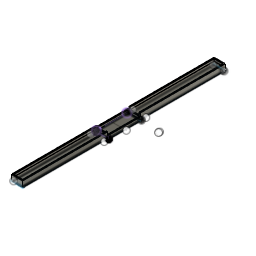
BitHolder (Autodesk Fusion 360 design; units mm, degrees)
Autodesk Fusion 360 part; units mm, degrees
sketch "Sketch2" plane through (0, 0, 0) normal (0, 0, 1) x (1, 0, 0)
  line L0 (0, 0) -> (25.146, 0)
  line L1 (25.146, 0) -> (25.146, 68.58)
  line L2 (25.146, 68.58) -> (0, 68.58)
  line L3 (0, 68.58) -> (0, 0)
  line L4 (0, 68.58) -> (-2.54, 68.58)
  line L5 (-2.54, 68.58) -> (-2.54, 0)
  line L6 (-2.54, 0) -> (0, 0)
  line L7 (0, 0) -> (0, 68.58)
  line L8 (25.146, 0) -> (27.686, 0)
  line L9 (27.686, 0) -> (27.686, 68.58)
  line L10 (27.686, 68.58) -> (25.146, 68.58)
  line L11 (25.146, 68.58) -> (25.146, 0)
  line L12 (71.12, 68.58) -> (71.12, 66.04)
  line L13 (-2.54, 66.04) -> (-2.54, 68.58)
  line L14 (-2.54, 68.58) -> (27.686, 68.58)
  line L15 (27.686, 68.58) -> (27.686, 71.12)
  line L16 (27.686, 71.12) -> (-2.54, 71.12)
  line L17 (-2.54, 71.12) -> (-2.54, 68.58)
  line L18 (27.686, 0) -> (-2.54, 0)
  line L19 (-2.54, 0) -> (-2.54, -2.54)
  line L20 (-2.54, -2.54) -> (27.686, -2.54)
  line L21 (27.686, -2.54) -> (27.686, 0)
  dimension "d46" = 25.146
  dimension "d47" = 68.58
  dimension "d48" = 2.54
  dimension "d49" = 2.54
  dimension "d51" = 2.54
  dimension "d52" = 2.54
  dimension "d53" = 30.226
  dimension "d54" = 2.54
  dimension "d55" = 30.226
  constraint horizontal L0
  constraint vertical L1
  constraint horizontal L2
  constraint vertical L3
  constraint coincident L0.start L3.end
  constraint horizontal L4
  constraint vertical L5
  constraint horizontal L6
  constraint vertical L7
  constraint horizontal L8
  constraint vertical L9
  constraint horizontal L10
  constraint vertical L11
  constraint vertical L12
  constraint vertical L13
  constraint horizontal L14
  constraint vertical L15
  constraint horizontal L16
  constraint vertical L17
  constraint horizontal L18
  constraint vertical L19
  constraint horizontal L20
  constraint vertical L21
  measures "d46" distance of L1.end L2.end
  measures "d47" distance of L0.start L2.end
  measures "d48" distance of L2.end L4.end
  measures "d49" distance of L9.end L1.end
  measures "d51" distance of L4.end L13.start
  measures "d52" distance of L4.end L16.end
  measures "d53" distance of L8.end L5.end
  measures "d54" distance of L5.end L19.end
  measures "d55" distance of L15.end L16.end
extrude "Extrude10" add sketch "Sketch2" along normal blind 2.54 contours L0 L1 L2 L3 L7 L11 L14 L18 makes body 1
extrude "Extrude11" add sketch "Sketch2" along normal blind 7.62 contours L1 L8 L9 L10 L11 L14 L18 bodies 1
extrude "Extrude12" add sketch "Sketch2" along normal blind 7.62 contours L0 L6 L8 L18 L19 L20 L21 bodies 1
extrude "Extrude13" add sketch "Sketch2" along normal blind 7.62 contours L3 L4 L5 L6 L7 L13 L14 L18 bodies 1
extrude "Extrude14" add sketch "Sketch2" along normal blind 7.62 contours L2 L4 L10 L14 L15 L16 L17 bodies 1
sketch "Sketch3" plane through (0, 0, 0) normal (0, 0, 1) x (1, 0, 0)
  line L0 (2.573, -2.54) -> (22.573, -2.54)
  line L1 (22.573, -2.54) -> (22.573, -191.036)
  line L2 (22.573, -191.036) -> (2.573, -191.036)
  line L3 (2.573, -191.036) -> (2.573, -2.54)
  line L4 (-2.54, -2.54) -> (27.686, -2.54)
  line L5 (27.686, -2.54) -> (27.686, -12.7) construction
  line L6 (-2.54, -2.54) -> (-2.54, -13.5317) construction
  line L7 (2.573, -2.54) -> (0.033, -2.54) construction
  line L8 (0.033, -191.036) -> (2.573, -191.036) construction
  line L9 (2.573, -2.54) -> (0.033, -2.54)
  line L10 (0.033, -2.54) -> (0.033, -191.036)
  line L11 (0.033, -191.036) -> (2.573, -191.036)
  line L12 (2.573, -191.036) -> (2.573, -2.54)
  line L13 (22.573, -2.54) -> (25.113, -2.54)
  line L14 (25.113, -2.54) -> (25.113, -191.036)
  line L15 (25.113, -191.036) -> (22.573, -191.036)
  line L16 (22.573, -191.036) -> (22.573, -2.54)
  line L17 (0.033, -191.036) -> (25.113, -191.036)
  line L18 (25.113, -191.036) -> (25.113, -193.576)
  line L19 (25.113, -193.576) -> (0.033, -193.576)
  line L20 (0.033, -193.576) -> (0.033, -191.036)
  line L21 (-2.54, 68.58) -> (-2.54, 0)
  line L22 (-2.54, 34.29) -> (30.48, 34.29)
  line L23 (25.113, 71.12) -> (25.113, 259.616)
  line L24 (22.573, 259.616) -> (22.573, 71.12)
  line L25 (2.573, 259.616) -> (2.573, 71.12)
  line L26 (0.033, 71.12) -> (0.033, 259.616)
  line L27 (2.573, 71.12) -> (22.573, 71.12)
  line L28 (2.573, 71.12) -> (0.033, 71.12)
  line L29 (22.573, 71.12) -> (25.113, 71.12)
  line L30 (27.686, 71.12) -> (27.686, 81.28) construction
  line L31 (-2.54, 71.12) -> (-2.54, 82.1117) construction
  line L32 (25.113, 262.156) -> (0.033, 262.156)
  line L33 (0.033, 259.616) -> (2.573, 259.616)
  line L34 (22.573, 259.616) -> (2.573, 259.616)
  line L35 (25.113, 259.616) -> (22.573, 259.616)
  line L36 (25.113, 259.616) -> (25.113, 262.156)
  line L37 (0.033, 262.156) -> (0.033, 259.616)
  dimension "d66" = 188.496
  dimension "d67" = 20
  dimension "d68" = 5.113
  dimension "d69" = 5.113
  dimension "d71" = 188.496
  dimension "d72" = 2.54
  dimension "d73" = 188.496
  dimension "d74" = 2.54
  dimension "d75" = 188.496
  dimension "d76" = 25.08
  dimension "d77" = 2.54
  constraint horizontal L0
  constraint vertical L1
  constraint horizontal L2
  constraint vertical L3
  constraint coincident L0.start L4
  constraint coincident L4.end L5.start
  constraint perpendicular L4 L5
  constraint coincident L4.start L6.start
  constraint perpendicular L4 L6
  constraint horizontal L7
  constraint horizontal L8
  constraint horizontal L9
  constraint vertical L10
  constraint horizontal L11
  constraint vertical L12
  constraint horizontal L13
  constraint vertical L14
  constraint horizontal L15
  constraint vertical L16
  constraint horizontal L17
  constraint vertical L18
  constraint horizontal L19
  constraint vertical L20
  constraint midpoint L21 L22.start
  constraint perpendicular L6 L22
  constraint symmetric L0.start L22 L25.end
  constraint symmetric L0.end L22 L24.end
  constraint symmetric L1.end L22 L24.start
  constraint symmetric L2.end L22 L25.start
  constraint symmetric L4.end L22 L30.start
  constraint symmetric L5.end L22 L30.end
  constraint symmetric L4.start L22 L31.start
  constraint symmetric L6.end L22 L31.end
  constraint symmetric L8.start L22 L26.end
  constraint symmetric L7.end L22 L26.start
  constraint symmetric L13.end L22 L23.start
  constraint symmetric L14.end L22 L23.end
  constraint symmetric L18.end L22 L32.start
  constraint symmetric L19.end L22 L32.end
  measures "d66" distance of L0.start L2.end
  measures "d67" distance of L1 L3
  measures "d68" distance of L3 L6
  measures "d69" distance of L1 L5
  measures "d71" distance of L0.start L2.end
  measures "d72" distance of L0.start L7.end
  measures "d73" distance of L0.start L2.end
  measures "d74" distance of L0.end L13.end
  measures "d75" distance of L0.end L1.end
  measures "d76" distance of L8.start L14.end
  measures "d77" distance of L8.start L19.end
extrude "Extrude15" add sketch "Sketch3" along normal blind 7.874 separate body contours L0 L1 L2 L3 L4 L12 L16 L17 makes body 2
extrude "Extrude16" add sketch "Sketch3" along normal blind 12.954 separate body contours L1 L4 L13 L14 L15 L16 L17 makes body 3
extrude "Extrude17" add sketch "Sketch3" along normal blind 12.954 separate body contours L3 L4 L9 L10 L11 L12 L17 makes body 4
extrude "Extrude18" add sketch "Sketch3" along normal blind 12.954 separate body contours L2 L11 L15 L17 L18 L19 L20 makes body 5
combine "Combine1" operation add target body 2 tool bodies 5 4 3
extrude "Extrude19" add sketch "Sketch3" along normal blind 7.874 separate body contours L24 L25 L27 L34 makes body 6
extrude "Extrude20" add sketch "Sketch3" along normal blind 12.954 separate body contours L23 L24 L29 L35 makes body 7
extrude "Extrude21" add sketch "Sketch3" along normal blind 12.954 separate body contours L32 L33 L34 L35 L36 L37 makes body 8
extrude "Extrude22" add sketch "Sketch3" along normal blind 12.954 separate body contours L25 L26 L28 L33 makes body 9
combine "Combine2" operation add target body 9 tool bodies 7 6 8
equation "ReaderDepth = 0.9 in"
equation "ReaderWidth = 0.9 in"
equation "Width = ReaderWidth * 3"
equation "Depth = ReaderDepth * 1.1"
equation "WallWidth = 0.1 in"
equation "BitHeight = 0.6 in"
equation "Height = 0.1 in"
equation "WallHeight = ( BitHeight / 3 ) + Height"
equation "RackLength = 188.496 mm"
equation "RackWidth = 20 mm"
equation "d46 = Depth"
equation "d47 = Width"
equation "d48 = WallWidth"
equation "d49 = WallWidth"
equation "d51 = WallWidth"
equation "d52 = WallWidth"
equation "d53 = Depth + ( 2 * WallWidth )"
equation "d54 = WallWidth"
equation "d55 = Depth + ( 2 * WallWidth )"
equation "d56 = Height"
equation "d58 = WallHeight"
equation "d60 = WallHeight"
equation "d62 = WallHeight"
equation "d64 = WallHeight"
equation "d66 = RackLength"
equation "d67 = RackWidth"
equation "d68 = d69"
equation "d71 = RackLength"
equation "d72 = WallWidth"
equation "d73 = RackLength"
equation "d74 = WallWidth"
equation "d75 = RackLength"
equation "d76 = RackWidth + ( 2 * WallWidth )"
equation "d77 = WallWidth"
equation "RackHolderHeight = 0.31 in"
equation "RackHolderWalls = RackHolderHeight + ( WallHeight - Height )"
equation "d80 = RackHolderHeight"
equation "d82 = RackHolderWalls"
equation "d84 = RackHolderWalls"
equation "d86 = RackHolderWalls"
equation "d88 = RackHolderHeight"
equation "d90 = RackHolderWalls"
equation "d92 = RackHolderWalls"
equation "d94 = RackHolderWalls"
